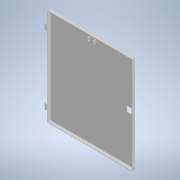
# Autodesk Inventor part: jJBDOOR161410HC1
Saved by Autodesk Inventor 2021 (Build 250183000, 183)
## iProperties
Created: 2025-08-10
Part Number: jJBDOOR161410HC1
Material: Generic
Catalog Web Link: www.cadenas.de
Description: JB DOOR-JB
Vendor: RITTAL
Document SubType Name: Modeling
Designer: psAdmin
Manufacturer: RITTAL
Mass: 306.751 g
Surface Area: 3200.97 cm^2
Volume: 306.751 cm^3
Density: 1 g/cm^3
Appearance: PSOLRGB-175-175-175
Category: PARTsolutions
Company: RITTAL
Title: jJBDOOR161410HC1
Author: Cadenas PARTsolutions
Comments: JB
PSOL_IDENT_0: {$CADENAS_DATA/23d-libs/rittal/schaltschranksys/kleingeh/jb_parts/jb_door.prj},186 {VTYP=3D},{NB=jJB
PSOL_IDENT_1: DOOR161410HC1},{LINA=jJBDOOR161410HC1},{NN=JB DOOR},{DATE=20.08.2024 09:27:20},{GEOMDATE=14.07.2022
PSOL_IDENT_2: 11:29:00},{VERSION=},{LINEID=190},{WBVAR=DETAIL},{WBNUMERIC=DETAIL}  {NB=jJBDOOR161410HC1},{LINA=jJB
PSOL_IDENT_3: DOOR161410HC1},{KT=DUMMY},{PN=161410HC},{H=400.00000},{B=350.00000},{T=15.00000},{DETAIL=1},{SPOSY=1
PSOL_IDENT_4: 66.75000},{THP=142.20000},{LHP=142.20000},{NOH=2},{MT=cs},{GS=0.00000},{X=0.13000}
NB: jJBDOOR161410HC1
NN: JB DOOR
NT: JB
NBSYN: jJBDOOR$PN.$DETAIL.
LINA: jJBDOOR161410HC1
CATALOG: Rittal
PN: 161410HC
H: 400
B: 350
T: 15
DETAIL: High
SPOSY: 166.75
THP: 142.2
LHP: 142.2
NOH: 2
MT: cs
GS: 0
X: 0.13
SUPPLIER: RITTAL
ARTICLENO: jJBDOOR161410HC1
BOMINFO: jJBDOOR161410HC1
CREATOR: CADENAS GmbH
Autodesk Inventor part; units mm, degrees
sketch "Sketch_2" plane through (0, 0, 0) normal (0, 0, 1) x (1, 0, 0)
  arc A0 (-175, -195) -> (-170, -200) centre (-170, -195) ccw
  line L0 (-170, -200) -> (170, -200)
  arc A1 (170, -200) -> (175, -195) centre (170, -195) ccw
  line L1 (175, -195) -> (175, 195)
  arc A2 (175, 195) -> (170, 200) centre (170, 195) ccw
  line L2 (170, 200) -> (-170, 200)
  arc A3 (-170, 200) -> (-175, 195) centre (-170, 195) ccw
  line L3 (-175, 195) -> (-175, -195)
  constraints: 8 end point, 8 point on circle, 4 centre point
extrude "Extrusion1" add sketch "Sketch_2" along normal blind 15
sketch "Sketch_3" plane through (0, 0, 0) normal (0, 1, 0) x (-1, 0, 0)
  line L0 (350, -15) -> (350, 30)
  line L1 (350, 30) -> (-350, 30)
  line L2 (-350, 30) -> (-350, -15)
  line L3 (-350, -15) -> (350, -15)
  line L4 (175, 5) -> (175, 15)
  line L5 (175, 15) -> (-175, 15)
  line L6 (-175, 15) -> (-175, 5)
  arc A0 (-175, 5) -> (-170, 0) centre (-170, 5) ccw
  line L7 (-170, 0) -> (170, 0)
  arc A1 (170, 0) -> (175, 5) centre (170, 5) ccw
  constraints: 16 end point, 4 point on circle, 2 centre point
extrude "Extrusion2" cut sketch "Sketch_3" along normal mid plane 400
sketch "Sketch_4" plane through (0, 0, 0) normal (1, 0, 0) x (0, 1, 0)
  line L0 (400, 30) -> (-400, 30)
  line L1 (-400, 30) -> (-400, -15)
  line L2 (-400, -15) -> (400, -15)
  line L3 (400, -15) -> (400, 30)
  line L4 (200, 15) -> (-200, 15)
  line L5 (-200, 15) -> (-200, 5)
  arc A0 (-200, 5) -> (-195, 0) centre (-195, 5) ccw
  line L6 (-195, 0) -> (195, 0)
  arc A1 (195, 0) -> (200, 5) centre (195, 5) ccw
  line L7 (200, 5) -> (200, 15)
  constraints: 16 end point, 4 point on circle, 2 centre point
extrude "Extrusion3" cut sketch "Sketch_4" along normal mid plane 350
sketch "Sketch_8" plane through (0, 0, 2) normal (0, 0, 1) x (1, 0, 0)
  arc A0 (-173.25, -194.75) -> (-169.75, -198.25) centre (-169.75, -194.75) ccw
  line L0 (-169.75, -198.25) -> (169.75, -198.25)
  arc A1 (169.75, -198.25) -> (173.25, -194.75) centre (169.75, -194.75) ccw
  line L1 (173.25, -194.75) -> (173.25, 194.75)
  arc A2 (173.25, 194.75) -> (169.75, 198.25) centre (169.75, 194.75) ccw
  line L2 (169.75, 198.25) -> (-169.75, 198.25)
  arc A3 (-169.75, 198.25) -> (-173.25, 194.75) centre (-169.75, 194.75) ccw
  line L3 (-173.25, 194.75) -> (-173.25, -194.75)
  constraints: 8 end point, 8 point on circle, 4 centre point
extrude "Extrusion4" cut sketch "Sketch_8" along normal blind 15.5
sketch "Sketch_6" plane through (0, 0, 0) normal (0, 0, 1) x (1, 0, 0)
  line L0 (139.4, 11.05) -> (139.4, -11.05)
  line L1 (139.4, -11.05) -> (161.5, -11.05)
  line L2 (161.5, -11.05) -> (161.5, 11.05)
  line L3 (161.5, 11.05) -> (139.4, 11.05)
  constraints: 8 end point
extrude "Extrusion5" cut sketch "Sketch_6" along normal blind 3
sketch "Sketch_9" plane through (0, 166.75, 0) normal (0, 1, 0) x (1, 0, 0)
  line L0 (-12.5, -3.78) -> (-12.5, -14.5)
  line L1 (-12.5, -14.5) -> (-11, -14.5)
  line L2 (-11, -14.5) -> (-11, -3.78)
  arc A0 (-10.22, -3) -> (-11, -3.78) centre (-10.22, -3.78) ccw
  line L3 (-10.22, -3) -> (10.22, -3)
  arc A1 (11, -3.78) -> (10.22, -3) centre (10.22, -3.78) ccw
  line L4 (11, -3.78) -> (11, -14.5)
  line L5 (11, -14.5) -> (12.5, -14.5)
  line L6 (12.5, -14.5) -> (12.5, -3.78)
  arc A2 (12.5, -3.78) -> (10.22, -1.5) centre (10.22, -3.78) ccw
  line L7 (10.22, -1.5) -> (-10.22, -1.5)
  arc A3 (-10.22, -1.5) -> (-12.5, -3.78) centre (-10.22, -3.78) ccw
  constraints: 16 end point, 8 point on circle, 4 centre point
extrude "Extrusion6" add sketch "Sketch_9" along normal blind 17.25
sketch "Sketch_10" plane through (0, 0, 0) normal (1, 0, 0) x (0, 1, 0)
  line L0 (188.375, 20.7) -> (162.375, 20.7)
  line L1 (162.375, 20.7) -> (162.375, 8.7)
  line L2 (162.375, 8.7) -> (166.75, 8.7)
  arc A0 (171.05, 13) -> (166.75, 8.7) centre (171.05, 8.7) ccw
  line L3 (171.05, 13) -> (179.7, 13)
  arc A1 (184, 8.7) -> (179.7, 13) centre (179.7, 8.7) ccw
  line L4 (184, 8.7) -> (188.375, 8.7)
  line L5 (188.375, 8.7) -> (188.375, 20.7)
  constraints: 12 end point, 4 point on circle, 2 centre point
extrude "Extrusion7" cut sketch "Sketch_10" along normal mid plane 30
sketch "Sketch_11" plane through (0, 0, 0) normal (1, 0, 0) x (0, 1, 0)
  circle A0 centre (175.375, 9.2) radius 3.1
  constraints: 1 centre point
extrude "Extrusion8" cut sketch "Sketch_11" along normal mid plane 30
sketch "Sketch_12" plane through (0, 142.2, 0) normal (0, 1, 0) x (1, 0, 0)
  arc A0 (-174.9697, -18.53) -> (-175.1968, -20.9799) centre (-177.51, -19.53) ccw
  line L0 (-175.1968, -20.9799) -> (-172.6754, -16.9572)
  arc A1 (-172.6754, -16.9572) -> (-172.37, -15.895) centre (-174.37, -15.895) ccw
  line L1 (-172.37, -15.895) -> (-172.37, -8.3)
  line L2 (-172.37, -8.3) -> (-173.37, -8.3)
  line L3 (-173.37, -8.3) -> (-173.37, -15.895)
  arc A2 (-173.5227, -16.4261) -> (-173.37, -15.895) centre (-174.37, -15.895) ccw
  line L4 (-173.5227, -16.4261) -> (-176.0442, -20.4488)
  arc A3 (-175.9002, -18.8963) -> (-176.0442, -20.4488) centre (-177.51, -19.53) ccw
  line L5 (-175.9002, -18.8963) -> (-174.9697, -18.53)
  constraints: 12 end point, 8 point on circle, 4 centre point
extrude "Extrusion9" add sketch "Sketch_12" along normal mid plane 21.75
sketch "Sketch_7" plane through (0, -142.2, 0) normal (0, 1, 0) x (1, 0, 0)
  arc A0 (-174.9697, -18.34) -> (-175.1968, -20.7899) centre (-177.51, -19.34) ccw
  line L0 (-175.1968, -20.7899) -> (-172.6754, -16.7672)
  arc A1 (-172.6754, -16.7672) -> (-172.37, -15.705) centre (-174.37, -15.705) ccw
  line L1 (-172.37, -15.705) -> (-172.37, -8.11)
  line L2 (-172.37, -8.11) -> (-173.37, -8.11)
  line L3 (-173.37, -8.11) -> (-173.37, -15.705)
  arc A2 (-173.5227, -16.2361) -> (-173.37, -15.705) centre (-174.37, -15.705) ccw
  line L4 (-173.5227, -16.2361) -> (-176.0442, -20.2588)
  arc A3 (-175.9002, -18.7063) -> (-176.0442, -20.2588) centre (-177.51, -19.34) ccw
  line L5 (-175.9002, -18.7063) -> (-174.9697, -18.34)
  constraints: 12 end point, 8 point on circle, 4 centre point
extrude "Extrusion10" add sketch "Sketch_7" along normal mid plane 21.75
ref_plane "door_to_hinge_XY" through (-177.51, 142.2, 19.53) normal (0, 1, 0) x (1, 0, 0)
ref_plane "door_to_hinge_YZ" through (-177.51, 142.2, 19.53) normal (1, 0, 0) x (0, 0, -1)
ref_plane "door_to_hinge_ZX" through (-177.51, 142.2, 19.53) normal (0, 0, -1) x (0, 1, 0)
ref_plane "lock_XY" through (152.45, 0, -7) normal (0, 0, 1) x (1, 0, 0)
ref_plane "lock_YZ" through (152.45, 0, -7) normal (1, 0, 0) x (0, 1, 0)
ref_plane "lock_ZX" through (152.45, 0, -7) normal (0, 1, 0) x (0, 0, 1)
body "Solid1"
